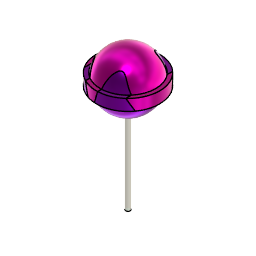
Lollipop (Autodesk Fusion 360 design; units mm, degrees)
part number: 2026-06-09-17-03-47-144
Autodesk Fusion 360 part; units mm, degrees
sketch "Sketch1" plane through (0, 0, 0) normal (0, 1, 0) x (1, 0, 0)
  line L0 (0, 0) -> (2, 0)
  line L1 (2, 0) -> (2, -75)
  line L2 (2, -75) -> (0, -75)
  line L3 (0, -75) -> (0, 0)
  arc A0 (0, -125) -> (0, -75) centre (0, -100) ccw
  line L4 (0.0011, -104.9159) -> (28.0011, -104.9159)
  line L5 (28.0011, -104.9159) -> (28.0011, -94.9159)
  line L6 (28.0011, -94.9159) -> (0.0011, -94.9159)
  line L7 (0.0011, -94.9159) -> (0.0011, -104.9159)
  line L8 (0, -125) -> (0, -75)
  dimension "d2" = 2
  dimension "d3" = 75
  dimension "d6" = 25
  dimension "d7" = 10
  dimension "d8" = 28
  constraint horizontal L0
  constraint vertical L1
  constraint horizontal L2
  constraint vertical L3
  constraint coincident L0.start L3.end
  constraint horizontal L4
  constraint vertical L5
  constraint horizontal L6
  constraint vertical L7
  constraint perpendicular L2 L8
  measures "d2" distance of L1 L3
  measures "d3" distance of L0.start L2.end
  measures "d6" radius of A0
  measures "d7" distance of L4 L6
  measures "d8" distance of L5 L7
revolve "Revolve1" add sketch "Sketch1" angle 360 about axis through (0, 0, 75) along (0, 0, -1)
sketch "Sketch2" plane through (0, 0, 0) normal (0, 1, 0) x (1, 0, 0)
  spline S0 degree 5 poles (-27.5301, -83.1039) (-27.0628, -86.263) (-26.1246, -92.1589) (-24.7065, -99.7366) (-22.794, -107.2971) (-20.3697, -112.5368) (-17.9202, -113.7525) (-15.4632, -111.4111) (-13.0288, -106.3632) (-10.6644, -100.0155) (-8.4224, -94.0586) (-6.3414, -90.0828) (-4.4314, -89.2595) (-2.6534, -91.9243) (-0.9119, -97.3928) (0.9197, -104.375) (2.9788, -111.2754) (5.3934, -116.5055) (8.2578, -118.8483) (11.6253, -117.5835) (15.5221, -112.3182) (19.0691, -104.7857) (21.9701, -97.2615) (24.0107, -91.4155) (25.0577, -88.285) knots 0 0 0 0 0 0 0.05 0.1 0.15 0.2 0.25 0.3 0.35 0.4 0.45 0.5 0.55 0.6 0.65 0.7 0.75 0.8 0.85 0.9 0.95 1 1 1 1 1 1
  point P0 (-15, -110)
  point P1 (-5, -90)
  point P2 (4.3334, -113.8017)
split_face "SplitFace1" 5 faces at (-11.8309, -20.4917, 108.0697) (27.862, -2.788, 101.5825) (26.6425, 2.6089, 104.9159) (-5.0241, -23.0704, 91.7834) (26.7224, 1.3911, 94.9159) by curves path "Sketch2" along S0
